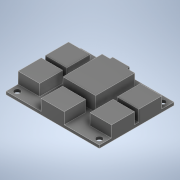
# Autodesk Inventor part: Quad-Load-Cell-Amplifier-to-RS-485-Conv-Module
Saved by Autodesk Inventor 2022.3 (Build 263350000, 350)
## iProperties
Created: 2023-04-23
Part Number: Quad-Load-Cell-Amplifier-to-RS-485-Conv-Module
Material: Generic
Document SubType Name: Modeling
Designer: Masato Kubotera
Density: 1 g/cm^3
Appearance: 滑らか - 黒
Author: Masato Kubotera
Autodesk Inventor part; units mm, degrees
ref_plane "YZ Plane" through (0, 0, 0) normal (1, 0, 0) x (0, 1, 0)
ref_plane "XZ Plane" through (0, 0, 0) normal (0, 1, 0) x (-1, 0, 0)
ref_plane "XY Plane" through (0, 0, 0) normal (0, 0, 1) x (1, 0, 0)
sketch "スケッチ1" plane through (0, 0, 0) normal (0, 0, 1) x (1, 0, 0)
  line L0 (-25, -20) -> (25, -20)
  line L1 (25, -20) -> (25, 20)
  line L2 (25, 20) -> (-25, 20)
  line L3 (-25, 20) -> (-25, -20)
  line L4 (-25, -20) -> (25, 20) construction
  line L5 (25, -20) -> (-25, 20) construction
  line L6 (-22, -17) -> (22, -17) construction
  line L7 (22, -17) -> (22, 17) construction
  line L8 (22, 17) -> (-22, 17) construction
  line L9 (-22, 17) -> (-22, -17) construction
  line L10 (-22, -17) -> (22, 17) construction
  line L11 (22, -17) -> (-22, 17) construction
  circle A0 centre (-22, -17) radius 1.6
  circle A1 centre (-22, 17) radius 1.6
  circle A2 centre (22, -17) radius 1.6
  circle A3 centre (22, 17) radius 1.6
  line L12 (-25, -13.5025) -> (-13.5, -13.5025)
  line L13 (-13.5, -13.5025) -> (-13.5, -1.1025)
  line L14 (-13.5, -1.1025) -> (-25, -1.1025)
  line L15 (-6.2, -20) -> (-6.2, -8.5)
  line L16 (-6.2, -8.5) -> (6.2, -8.5)
  line L17 (6.2, -8.5) -> (6.2, -20)
  line L18 (-25, 0) -> (25, 0) construction
  line L19 (0, -20) -> (0, 20) construction
  line L20 (-25, 13.5025) -> (-13.5, 13.5025)
  line L21 (-13.5, 13.5025) -> (-13.5, 1.1025)
  line L22 (-13.5, 1.1025) -> (-25, 1.1025)
  line L23 (25, -13.5025) -> (13.5, -13.5025)
  line L24 (13.5, -13.5025) -> (13.5, -1.1025)
  line L25 (13.5, -1.1025) -> (25, -1.1025)
  line L26 (13.5, 1.1025) -> (25, 1.1025)
  line L27 (13.5, 13.5025) -> (13.5, 1.1025)
  line L28 (25, 13.5025) -> (13.5, 13.5025)
  line L29 (-8.75, -5.76) -> (8.75, -5.76)
  line L30 (8.75, -5.76) -> (8.75, 15.24)
  line L31 (8.75, 15.24) -> (-8.75, 15.24)
  line L32 (-8.75, 15.24) -> (-8.75, -5.76)
  line L33 (-8.75, -5.76) -> (8.75, 15.24) construction
  line L34 (8.75, -5.76) -> (-8.75, 15.24) construction
  line L35 (-4.5, 15.24) -> (-4.5, 16.664)
  line L36 (-4.5, 16.664) -> (4.5, 16.664)
  line L37 (4.5, 16.664) -> (4.5, 15.24)
  point P0 (0, 0)
  point P1 (-13.5, -7.3025)
  point P2 (0, -8.5)
  point P3 (0, 4.74)
  point P4 (0, 16.664)
  point P5 (0, 4.74)
  dimension "d0" = 50
  dimension "d1" = 40
  dimension "d2" = 44
  dimension "d3" = 34
  dimension "d4" = 3.2
  dimension "d5" = 3.2
  dimension "d6" = 3.2
  dimension "d7" = 3.2
  dimension "d8" = 11.5
  dimension "d9" = 12.4
  dimension "d10" = 7.3025
  dimension "d11" = 11.5
  dimension "d12" = 12.4
  dimension "d17" = 17.5
  dimension "d18" = 21
  dimension "d19" = 9
  dimension "d20" = 1.424
  dimension "d21" = 15.26
  constraints: 76 end point, 14 midpoint, 12 symmetric about line, 11 perpendicular, 9 point on line, 6 parallel, 4 centre point, 4 coincident, 3 horizontal, 1 vertical
  measures "d0" distance of L2.end L1.end
  measures "d1" distance of L1.end L0.end
  measures "d2" distance of L8.end L7.end
  measures "d3" distance of L6.end L7.end
  measures "d4" diameter of A0
  measures "d5" diameter of A1
  measures "d6" diameter of A2
  measures "d7" diameter of A3
  measures "d8" distance of L12.start L12.end
  measures "d9" distance of L12.end L13.end
  measures "d10" distance from line of L18 point (-13.5, -7.303)
  measures "d11" distance of L15.start L15.end
  measures "d12" distance of L15.end L16.end
  measures "d17" distance of L31.end L30.end
  measures "d18" distance of L30.end L29.end
  measures "d19" distance of L35.end L36.end
  measures "d20" distance of L35.start L35.end
  measures "d21" distance of L19.end point (0, 4.74)
extrude "押し出し1" add sketch "スケッチ1" along normal blind 1.6 contours L3 L12 L13 L14 L22 L21 L20 L2 L1 L28 L27 L26 L25 L24 L23 L0 L17 L16 L15 | L15 L16 L17 L0 | L3 L14 L13 L12 | L3 L20 L21 L22 | L23 L24 L25 L1 | L26 L27 L28 L1 | L32 L31 L30 L29 | L35 L36 L37 L31
extrude "押し出し2" add sketch "スケッチ1" along normal blind 7.7 contours L15 L16 L17 L0 | L3 L14 L13 L12 | L3 L20 L21 L22 | L23 L24 L25 L1 | L26 L27 L28 L1
extrude "押し出し3" add sketch "スケッチ1" along normal blind 9.34 contours L32 L31 L30 L29 | L35 L36 L37 L31
equation "\"d5\" = d4"
equation "\"d6\" = d4"
equation "\"d7\" = d4"
equation "\"d11\" = d8"
equation "\"d12\" = d9"
